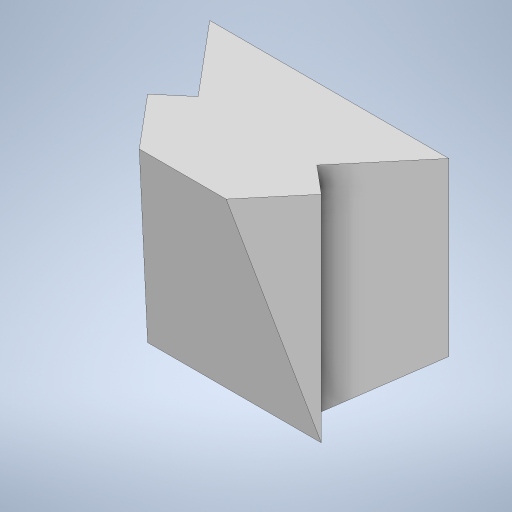
# Autodesk Inventor part: antana_middle_ex
Saved by Autodesk Inventor 2024.1 (Build 281209000, 209)
## iProperties
Created: 2024-02-25
Part Number: antana_middle_ex
Material: 一般
Document SubType Name: Modeling
Designer: hibik
Density: 1 g/cm^3
Appearance: 既定
Author: hibik
Autodesk Inventor part; units mm, degrees
ref_plane "YZ Plane" through (0, 0, 0) normal (1, 0, 0) x (0, 1, 0)
ref_plane "XZ Plane" through (0, 0, 0) normal (0, 1, 0) x (-1, 0, 0)
sketch "スケッチ1" plane through (0, 0, 0) normal (0, 0, 1) x (1, 0, 0)
  line L0 (-5, 9) -> (5, 9)
  line L1 (5, 9) -> (5, 0)
  line L2 (5, 0) -> (-5, 0)
  line L3 (-5, 0) -> (-5, 9)
  line L4 (-8.0749, 9) -> (-5, 9) construction
  point P0 (0, 0)
  point P1 (0, 9)
  point P2 (0, 0)
  dimension "d0" = 9
  dimension "d1" = 10
  dimension "d2" = 10
  constraints: 10 end point, 3 midpoint, 2 vertical alignment, 1 horizontal, 1 parallel, 1 perpendicular
  measures "d0" distance from line of L2.end L4
  measures "d1" distance of L0.start L0.end
  measures "d2" distance of L1.end L2.end
extrude "押し出し1" add sketch "スケッチ1" along normal blind 3
sketch "スケッチ2" plane through (-5, 9, 0) normal (0, 1, 0) x (1, 0, 0)
  line L0 (0, -3) -> (10, -3) projected
  line L1 (0, 0) -> (10, 0) projected
  line L2 (2.5173, -3) -> (0, 0)
  line L3 (10, 0) -> (7.4827, -3)
  line L4 (0, 0) -> (0, -3) projected
  line L5 (10, 0) -> (10, -3) projected
  point P0 (5, 0)
  dimension "d5" = 80
  dimension "d6" = 40
  dimension "d7" = 40
  constraints: 4 end point, 2 point on line
  measures "d5" angle of L3 L2
  measures "d6" angle of L4 L2
  measures "d7" angle of L5 L3
extrude "押し出し2" cut sketch "スケッチ2" against normal through all contours L4 L2 L0 | L3 L5 L0
sketch "スケッチ3" plane through (-5, 0, 0) normal (-0.7660444, 0, 0.6427876) x (0.6427876, 0, 0.7660444)
  line L0 (3.9162, 0) -> (0, 0) projected
  line L1 (3.9162, 9) -> (3.9162, 0) projected
  line L2 (0, 9) -> (3.9162, 9) projected
  line L3 (0, 9) -> (0, 0) projected
  line L4 (3.9162, 0) -> (7.1079, 0) projected
  line L5 (3.9162, 0) -> (-11.0838, 7)
  point P0 (3.2139, 0)
  point P1 (0, 1.8276)
  dimension "d10" = 15
  dimension "d11" = 7
  constraints: 2 end point
  measures "d10" distance from line of L1 L5.end
  measures "d11" distance from line of L0 L5.end
extrude "押し出し3" cut sketch "スケッチ3" against normal through all contours L0 L3 L5
sketch "スケッチ4" plane through (5, 0, 0) normal (0.7660444, 0, 0.6427876) x (0.6427876, 0, -0.7660444)
  line L0 (0, 0) -> (-3.9162, 0) projected
  line L1 (0, 0) -> (0, 9) projected
  line L2 (-3.9162, 9) -> (0, 9) projected
  line L3 (-3.9162, 0) -> (-3.9162, 9) projected
  line L4 (-3.9162, 0) -> (11.0838, 7)
  point P0 (-3.2139, 0)
  point P1 (0, 1.8276)
  dimension "d14" = 15
  dimension "d15" = 7
  constraints: 2 end point
  measures "d14" distance from line of L3 L4.end
  measures "d15" distance from line of L0 L4.end
extrude "押し出し4" cut sketch "スケッチ4" against normal through all contours L0 L4 L1
sketch "スケッチ5" plane through (0, 0, 3) normal (0, 0, 1) x (1, 0, 0)
  line L0 (-2.4827, 9) -> (-2.4827, 0) projected
  line L1 (-2.4827, 0) -> (2.4827, 0) projected
  line L2 (2.4827, 0) -> (2.4827, 9) projected
  line L3 (2.4827, 9) -> (-2.4827, 9) projected
  point P0 (0, 0)
extrude "押し出し5" add sketch "スケッチ5" along normal blind 10
sketch "スケッチ6" plane through (-2.4827, 0, 3) normal (-1, 0, 0) x (0, 0, 1)
  line L0 (0, 9) -> (0, 0) projected
  line L1 (0, 0) -> (10, 0) projected
  line L2 (10, 9) -> (10, 0) projected
  line L3 (0, 9) -> (10, 9) projected
  point P0 (-3, 0)
extrude "押し出し6" add sketch "スケッチ6" along normal blind 10
sketch "スケッチ7" plane through (2.4827, 0, 3) normal (1, 0, 0) x (0, 0, -1)
  line L0 (0, 0) -> (0, 9) projected
  line L1 (0, 9) -> (-10, 9) projected
  line L2 (-10, 0) -> (-10, 9) projected
  line L3 (0, 0) -> (-10, 0) projected
  point P0 (3, 0)
extrude "押し出し7" add sketch "スケッチ7" along normal blind 10
sketch "スケッチ8" plane through (5, 1.8276, 0) normal (0.7660444, 0, 0.6427876) x (0.6427876, 0, -0.7660444)
  line L0 (-7.1079, 7.1724) -> (-7.1079, -1.8276) projected
  line L1 (-3.9162, -1.8276) -> (0, 0) projected
  line L2 (0, 0) -> (0, 7.1724) projected
  line L3 (-3.9162, 7.1724) -> (0, 7.1724) projected
  line L4 (-3.9162, -1.8276) -> (-3.9162, 7.1724) projected
  line L5 (-3.9162, 20) -> (16.0838, 20)
  line L6 (16.0838, 20) -> (16.0838, -10)
  line L7 (16.0838, -10) -> (-3.9162, -10)
  line L8 (-3.9162, -10) -> (-3.9162, 20)
  point P0 (-3.2139, -1.8276)
  point P1 (-3.9162, -1.8276)
  point P2 (-3.9162, 7.1724)
  constraints: 8 end point, 2 parallel, 1 collinear, 1 horizontal, 1 perpendicular
extrude "押し出し8" cut sketch "スケッチ8" along normal through all
sketch "スケッチ9" plane through (-5, 1.8276, 0) normal (-0.7660444, 0, 0.6427876) x (0.6427876, 0, 0.7660444)
  line L0 (0, 0) -> (3.9162, -1.8276) projected
  line L1 (3.9162, 7.1724) -> (3.9162, -1.8276) projected
  line L2 (0, 7.1724) -> (3.9162, 7.1724) projected
  line L3 (0, 7.1724) -> (0, 0) projected
  line L4 (-16.0838, 20) -> (3.9162, 20)
  line L5 (3.9162, 20) -> (3.9162, -20)
  line L6 (3.9162, -20) -> (-16.0838, -20)
  line L7 (-16.0838, -20) -> (-16.0838, 20)
  point P0 (3.2139, -1.8276)
  point P1 (3.9162, 7.1724)
  point P2 (3.9162, -1.8276)
  constraints: 8 end point, 2 parallel, 1 collinear, 1 horizontal, 1 perpendicular
extrude "押し出し9" cut sketch "スケッチ9" along normal through all
sketch "スケッチ10" plane through (2.4827, 0, 3) normal (0.6427876, 0, -0.7660444) x (-0.7660444, 0, -0.6427876)
  line L0 (-13.0541, 9) -> (0, 9) projected
  line L1 (0, 0) -> (0, 9) projected
  line L2 (-1.5, 9) -> (0, 9)
  line L3 (0, 9) -> (0, 0)
  line L4 (0, 0) -> (-1.5, 0)
  line L5 (-1.5, 0) -> (-1.5, 9)
  line L6 (-13.0541, 9) -> (0, 9) projected
  line L7 (-13.0541, 0) -> (-13.0541, 9) projected
  line L8 (0, 0) -> (-13.0541, 0) projected
  line L9 (0, 0) -> (0, 9) projected
  line L10 (-20, 9) -> (-13.0541, 9)
  line L11 (-13.0541, 9) -> (-13.0541, 0)
  line L12 (-13.0541, 0) -> (-20, 0)
  line L13 (-20, 0) -> (-20, 9)
  line L14 (-13.0541, 0) -> (-13.0541, 9) projected
  line L15 (0, 0) -> (-13.0541, 0) projected
  point P0 (3.8302, 0)
  point P1 (-1.5, 0)
  dimension "d28" = 1.5
  constraints: 16 end point, 4 parallel, 3 collinear, 2 horizontal, 2 perpendicular, 1 point on line
  measures "d28" distance between parallel lines of L1 L5
extrude "押し出し10" cut sketch "スケッチ10" against normal through all contours L0 L5 L8 L7 | L7 L12 L13 L10
sketch "スケッチ11" plane through (-2.4827, 0, 3) normal (-0.6427876, 0, -0.7660444) x (-0.7660444, 0, 0.6427876)
  line L0 (-7.6604, 9) -> (0, 9) projected
  line L1 (-4.0642, 0) -> (7.552, 0) projected
  line L2 (0, 9) -> (1.5, 9)
  line L3 (1.5, 9) -> (1.5, 0)
  line L4 (1.5, 0) -> (0, 0)
  line L5 (0, 0) -> (0, 9)
  line L6 (1.5, 9) -> (20, 9)
  line L7 (20, 9) -> (20, 0)
  line L8 (20, 0) -> (1.5, 0)
  line L9 (1.5, 0) -> (1.5, 9)
  line L10 (13.0541, 0) -> (0, 0) projected
  point P0 (-3.8302, 0)
  dimension "d31" = 1.5
  constraints: 16 end point, 4 parallel, 2 horizontal, 2 perpendicular, 1 collinear, 1 point on line
  measures "d31" distance between parallel lines of L5 L3
extrude "押し出し11" cut sketch "スケッチ11" against normal through all contours L3 L6 L7 L8 L1
ref_plane "作業平面1" through (-1.8159, 9, 6.1283) normal (0, 0.2337903, -0.972287) x (1, 0, 0)
sketch "スケッチ12" plane through (-1.8159, 9, 6.1283) normal (0, 0.2337903, -0.972287) x (1, 0, 0)
  line L0 (-10, -6.5677) -> (20, -6.5677)
  line L1 (20, -6.5677) -> (20, 15.9547)
  line L2 (20, 15.9547) -> (-10, 15.9547)
  line L3 (-10, 15.9547) -> (-10, -6.5677)
  point P0 (1.8159, 10.1833)
  constraints: 8 end point, 2 parallel, 1 horizontal, 1 perpendicular
extrude "押し出し12" cut sketch "スケッチ12" against normal through all
equation "\"d6\" = d7"
